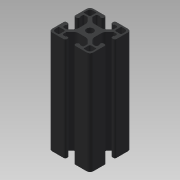
# Autodesk Inventor part: 40-4040-LITE-BLACK-FB
Saved by Autodesk Inventor 2013 (Build 170138000, 138)
## iProperties
Company: 80/20 Inc.
Created: 2014-04-23
Part Number: 40-4040-LITE-BLACK-FB
Material: Generic
Document SubType Name: Modeling
Designer: Ross Bowman
Density: 1 g/cm^3
Engineer: Ross Bowman
Catalog Web Link: 8020.net
Vendor: 80/20 Inc.
Material: 6105-T5 Aluminum
Author: Ross Bowman
Keywords: 80/20 , 8020 , T-Slot , Extrusion
Autodesk Inventor part; units mm, degrees
ref_plane "YZ Plane" through (0, 0, 0) normal (1, 0, 0) x (0, 1, 0)
ref_plane "XZ Plane" through (0, 0, 0) normal (0, 1, 0) x (-1, 0, 0)
ref_plane "XY Plane" through (0, 0, 0) normal (0, 0, 1) x (1, 0, 0)
sketch "Sketch1" plane through (0, 0, 0) normal (0, 0, 1) x (1, 0, 0)
  arc A0 (-15.55, 18.35) -> (-18.35, 15.55) centre (-15.55, 15.55) ccw
  line L0 (-12.57, 18.35) -> (-15.55, 18.35)
  arc A1 (-11.94, 17.72) -> (-12.57, 18.35) centre (-12.57, 17.72) ccw
  line L1 (-11.94, 13.21) -> (-11.94, 17.72)
  arc A2 (-13.21, 11.94) -> (-11.94, 13.21) centre (-13.21, 13.21) ccw
  line L2 (-17.72, 11.94) -> (-13.21, 11.94)
  arc A3 (-18.35, 12.57) -> (-17.72, 11.94) centre (-17.72, 12.57) ccw
  line L3 (-18.35, 15.55) -> (-18.35, 12.57)
  arc A4 (18.35, -12.57) -> (17.72, -11.94) centre (17.72, -12.57) ccw
  line L4 (18.35, -15.55) -> (18.35, -12.57)
  arc A5 (15.55, -18.35) -> (18.35, -15.55) centre (15.55, -15.55) ccw
  line L5 (12.57, -18.35) -> (15.55, -18.35)
  arc A6 (11.94, -17.72) -> (12.57, -18.35) centre (12.57, -17.72) ccw
  line L6 (11.94, -13.21) -> (11.94, -17.72)
  arc A7 (13.21, -11.94) -> (11.94, -13.21) centre (13.21, -13.21) ccw
  line L7 (17.72, -11.94) -> (13.21, -11.94)
  arc A8 (-18.35, -15.55) -> (-15.55, -18.35) centre (-15.55, -15.55) ccw
  line L8 (-18.35, -12.57) -> (-18.35, -15.55)
  arc A9 (-17.72, -11.94) -> (-18.35, -12.57) centre (-17.72, -12.57) ccw
  line L9 (-13.21, -11.94) -> (-17.72, -11.94)
  arc A10 (-11.94, -13.21) -> (-13.21, -11.94) centre (-13.21, -13.21) ccw
  line L10 (-11.94, -17.72) -> (-11.94, -13.21)
  arc A11 (-12.57, -18.35) -> (-11.94, -17.72) centre (-12.57, -17.72) ccw
  line L11 (-15.55, -18.35) -> (-12.57, -18.35)
  circle A12 centre (0, 0) radius 3.4
  arc A13 (18.35, 15.55) -> (15.55, 18.35) centre (15.55, 15.55) ccw
  line L12 (18.35, 12.57) -> (18.35, 15.55)
  arc A14 (17.72, 11.94) -> (18.35, 12.57) centre (17.72, 12.57) ccw
  line L13 (13.21, 11.94) -> (17.72, 11.94)
  arc A15 (11.94, 13.21) -> (13.21, 11.94) centre (13.21, 13.21) ccw
  line L14 (11.94, 17.72) -> (11.94, 13.21)
  arc A16 (12.57, 18.35) -> (11.94, 17.72) centre (12.57, 17.72) ccw
  line L15 (15.55, 18.35) -> (12.57, 18.35)
  arc A17 (7.685, -3.3582) -> (9.0741, -6.7149) centre (12.435, -3.3582) ccw
  line L16 (7.685, -3.3582) -> (7.685, 3.3582)
  arc A18 (9.0741, 6.7149) -> (7.685, 3.3582) centre (12.435, 3.3582) ccw
  line L17 (9.0741, 6.7149) -> (12.3735, 10.0183)
  arc A19 (13.0032, 10.2794) -> (12.3735, 10.0183) centre (13.0032, 9.3894) ccw
  line L18 (13.0032, 10.2794) -> (15.2988, 10.2794)
  arc A20 (16.5688, 9.0094) -> (15.2988, 10.2794) centre (15.2988, 9.0094) ccw
  line L19 (16.5688, 9.0094) -> (16.5688, 6.9014)
  line L20 (16.5688, 6.9014) -> (15.94, 6.9014)
  line L21 (15.94, 6.9014) -> (15.94, 5.7581)
  arc A21 (15.94, 5.7581) -> (17.51, 4.1881) centre (17.51, 5.7581) ccw
  line L22 (17.51, 4.1881) -> (18.43, 4.1881)
  arc A22 (18.43, 4.1881) -> (20, 5.7581) centre (18.43, 5.7581) ccw
  line L23 (20, 5.7581) -> (20, 16.83)
  arc A23 (20, 16.83) -> (16.83, 20) centre (16.83, 16.83) ccw
  line L24 (16.83, 20) -> (5.63, 20)
  arc A24 (5.63, 20) -> (4.06, 18.43) centre (5.63, 18.43) ccw
  line L25 (4.06, 18.43) -> (4.06, 17.6962)
  arc A25 (4.06, 17.6962) -> (5.63, 16.1262) centre (5.63, 17.6962) ccw
  line L26 (5.63, 16.1262) -> (6.7839, 16.1262)
  line L27 (6.7839, 16.1262) -> (6.7839, 16.8867)
  line L28 (6.7839, 16.8867) -> (9.015, 16.8867)
  arc A26 (10.285, 15.6167) -> (9.015, 16.8867) centre (9.015, 15.6167) ccw
  line L29 (10.285, 15.6167) -> (10.285, 12.9222)
  arc A27 (10.1664, 12.4784) -> (10.285, 12.9222) centre (9.395, 12.9222) ccw
  line L30 (10.1664, 12.4784) -> (6.7706, 9.0783)
  arc A28 (3.4098, 7.685) -> (6.7706, 9.0783) centre (3.4098, 12.435) ccw
  line L31 (3.4098, 7.685) -> (-3.4098, 7.685)
  arc A29 (-6.7706, 9.0783) -> (-3.4098, 7.685) centre (-3.4098, 12.435) ccw
  line L32 (-6.7706, 9.0783) -> (-10.1664, 12.4784)
  arc A30 (-10.285, 12.9222) -> (-10.1664, 12.4784) centre (-9.395, 12.9222) ccw
  line L33 (-10.285, 12.9222) -> (-10.285, 15.6167)
  arc A31 (-9.015, 16.8867) -> (-10.285, 15.6167) centre (-9.015, 15.6167) ccw
  line L34 (-9.015, 16.8867) -> (-6.7839, 16.8867)
  line L35 (-6.7839, 16.8867) -> (-6.7839, 16.1262)
  line L36 (-6.7839, 16.1262) -> (-5.63, 16.1262)
  arc A32 (-5.63, 16.1262) -> (-4.06, 17.6962) centre (-5.63, 17.6962) ccw
  line L37 (-4.06, 17.6962) -> (-4.06, 18.43)
  arc A33 (-4.06, 18.43) -> (-5.63, 20) centre (-5.63, 18.43) ccw
  line L38 (-5.63, 20) -> (-16.83, 20)
  arc A34 (-16.83, 20) -> (-20, 16.83) centre (-16.83, 16.83) ccw
  line L39 (-20, 16.83) -> (-20, 5.7581)
  arc A35 (-20, 5.7581) -> (-18.43, 4.1881) centre (-18.43, 5.7581) ccw
  line L40 (-18.43, 4.1881) -> (-17.51, 4.1881)
  arc A36 (-17.51, 4.1881) -> (-15.94, 5.7581) centre (-17.51, 5.7581) ccw
  line L41 (-15.94, 5.7581) -> (-15.94, 6.9014)
  line L42 (-15.94, 6.9014) -> (-16.5688, 6.9014)
  line L43 (-16.5688, 6.9014) -> (-16.5688, 9.0094)
  arc A37 (-15.2988, 10.2794) -> (-16.5688, 9.0094) centre (-15.2988, 9.0094) ccw
  line L44 (-15.2988, 10.2794) -> (-13.0032, 10.2794)
  arc A38 (-12.3735, 10.0183) -> (-13.0032, 10.2794) centre (-13.0032, 9.3894) ccw
  line L45 (-12.3735, 10.0183) -> (-9.0741, 6.7149)
  arc A39 (-7.685, 3.3582) -> (-9.0741, 6.7149) centre (-12.435, 3.3582) ccw
  line L46 (-7.685, 3.3582) -> (-7.685, -3.3582)
  arc A40 (-9.0741, -6.7149) -> (-7.685, -3.3582) centre (-12.435, -3.3582) ccw
  line L47 (-9.0741, -6.7149) -> (-12.3735, -10.0183)
  arc A41 (-13.0032, -10.2794) -> (-12.3735, -10.0183) centre (-13.0032, -9.3894) ccw
  line L48 (-13.0032, -10.2794) -> (-15.2988, -10.2794)
  arc A42 (-16.5688, -9.0094) -> (-15.2988, -10.2794) centre (-15.2988, -9.0094) ccw
  line L49 (-16.5688, -9.0094) -> (-16.5688, -6.9014)
  line L50 (-16.5688, -6.9014) -> (-15.94, -6.9014)
  line L51 (-15.94, -6.9014) -> (-15.94, -5.7581)
  arc A43 (-15.94, -5.7581) -> (-17.51, -4.1881) centre (-17.51, -5.7581) ccw
  line L52 (-17.51, -4.1881) -> (-18.43, -4.1881)
  arc A44 (-18.43, -4.1881) -> (-20, -5.7581) centre (-18.43, -5.7581) ccw
  line L53 (-20, -5.7581) -> (-20, -16.83)
  arc A45 (-20, -16.83) -> (-16.83, -20) centre (-16.83, -16.83) ccw
  line L54 (-16.83, -20) -> (-5.63, -20)
  arc A46 (-5.63, -20) -> (-4.06, -18.43) centre (-5.63, -18.43) ccw
  line L55 (-4.06, -18.43) -> (-4.06, -17.6962)
  arc A47 (-4.06, -17.6962) -> (-5.63, -16.1262) centre (-5.63, -17.6962) ccw
  line L56 (-5.63, -16.1262) -> (-6.7839, -16.1262)
  line L57 (-6.7839, -16.1262) -> (-6.7839, -16.8867)
  line L58 (-6.7839, -16.8867) -> (-9.015, -16.8867)
  arc A48 (-10.285, -15.6167) -> (-9.015, -16.8867) centre (-9.015, -15.6167) ccw
  line L59 (-10.285, -15.6167) -> (-10.285, -12.9222)
  arc A49 (-10.1664, -12.4784) -> (-10.285, -12.9222) centre (-9.395, -12.9222) ccw
  line L60 (-10.1664, -12.4784) -> (-6.7706, -9.0783)
  arc A50 (-3.4098, -7.685) -> (-6.7706, -9.0783) centre (-3.4098, -12.435) ccw
  line L61 (-3.4098, -7.685) -> (3.4098, -7.685)
  arc A51 (6.7706, -9.0783) -> (3.4098, -7.685) centre (3.4098, -12.435) ccw
  line L62 (6.7706, -9.0783) -> (10.1664, -12.4784)
  arc A52 (10.285, -12.9222) -> (10.1664, -12.4784) centre (9.395, -12.9222) ccw
  line L63 (10.285, -12.9222) -> (10.285, -15.6167)
  arc A53 (9.015, -16.8867) -> (10.285, -15.6167) centre (9.015, -15.6167) ccw
  line L64 (9.015, -16.8867) -> (6.7839, -16.8867)
  line L65 (6.7839, -16.8867) -> (6.7839, -16.1262)
  line L66 (6.7839, -16.1262) -> (5.63, -16.1262)
  arc A54 (5.63, -16.1262) -> (4.06, -17.6962) centre (5.63, -17.6962) ccw
  line L67 (4.06, -17.6962) -> (4.06, -18.43)
  arc A55 (4.06, -18.43) -> (5.63, -20) centre (5.63, -18.43) ccw
  line L68 (5.63, -20) -> (16.83, -20)
  arc A56 (16.83, -20) -> (20, -16.83) centre (16.83, -16.83) ccw
  line L69 (20, -16.83) -> (20, -5.7581)
  arc A57 (20, -5.7581) -> (18.43, -4.1881) centre (18.43, -5.7581) ccw
  line L70 (18.43, -4.1881) -> (17.51, -4.1881)
  arc A58 (17.51, -4.1881) -> (15.94, -5.7581) centre (17.51, -5.7581) ccw
  line L71 (15.94, -5.7581) -> (15.94, -6.9014)
  line L72 (15.94, -6.9014) -> (16.5688, -6.9014)
  line L73 (16.5688, -6.9014) -> (16.5688, -9.0094)
  arc A59 (15.2988, -10.2794) -> (16.5688, -9.0094) centre (15.2988, -9.0094) ccw
  line L74 (15.2988, -10.2794) -> (13.0032, -10.2794)
  arc A60 (12.3735, -10.0183) -> (13.0032, -10.2794) centre (13.0032, -9.3894) ccw
  line L75 (12.3735, -10.0183) -> (9.0741, -6.7149)
  constraints: 152 end point, 120 point on circle, 61 centre point
extrude "Extrusion1" add sketch "Sketch1" against normal blind 100
body "Solid1"
